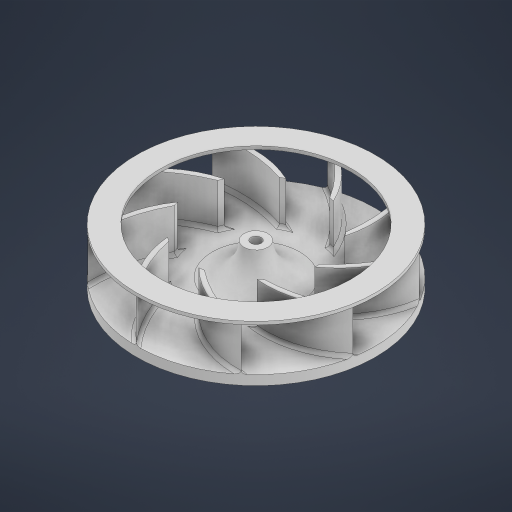
# Autodesk Inventor part: Fan4
Saved by Autodesk Inventor 2023 (Build 270158000, 158)
## iProperties
Created: 2022-10-05
Part Number: Fan4
Material: 一般
Document SubType Name: Modeling
Designer: neko2
Density: 1 g/cm^3
Appearance: 既定
Author: neko2
Autodesk Inventor part; units mm, degrees
ref_plane "YZ Plane" through (0, 0, 0) normal (1, 0, 0) x (0, 1, 0)
ref_plane "XZ Plane" through (0, 0, 0) normal (0, 1, 0) x (-1, 0, 0)
ref_plane "XY Plane" through (0, 0, 0) normal (0, 0, 1) x (1, 0, 0)
sketch "スケッチ1" plane through (0, 0, 0) normal (0, 1, 0) x (-1, 0, 0)
  circle A0 centre (0, 0) radius 7.5
  dimension "d0" = 15
  constraints: 1 centre point, 1 coincident
  measures "d0" diameter of A0
extrude "押し出し1" add sketch "スケッチ1" along normal blind 0.6
sketch "スケッチ2" plane through (0, 0.6, 0) normal (0, 1, 0) x (1, 0, 0)
  circle A0 centre (0, 0) radius 7.5 projected
  circle A1 centre (0, 0) radius 4
  arc A2 (-2, -3.4641) -> (0, -7.5) centre (6.8076, -1.613) ccw
  arc A3 (-2.254, -3.3045) -> (0, -7.5) centre (3.7244, -2.7959) ccw
  dimension "d27" = 8
  dimension "d30" = 9
  dimension "d31" = 6
  dimension "d32" = 0.3
  dimension "d33" = 2
  constraints: 6 point on circle, 3 centre point, 2 vertical alignment, 1 coincident, 1 other
  measures "d27" diameter of A1
  measures "d30" radius of A2
  measures "d31" radius of A3
  measures "d32" distance of A1.start A1.end
  measures "d33" horizontal distance of point (0, 0) A1.start
extrude "押し出し2" add sketch "スケッチ2" along normal blind 2.7 contours A3 A1 A2
fillet "フィレット2" radius 0.2 3 edges at (-1.5611, 0.6, 5.6355) (-1.2566, 0.6, 5.6092) (-2.1285, 0.6, 3.3867)
pattern_circular "円形状パターン3" count 9 over 360 about axis through (0, -10, 0) along (0, 1, 0)
sketch "スケッチ6" plane through (-4.456, 3.3, -1.3534) normal (0, 1, 0) x (0.7460152, 0, 0.665929)
  circle A0 centre (4.2256, 1.9577) radius 6
  circle A1 centre (4.2256, 1.9577) radius 7.5 projected
  circle A2 centre (4.2256, 1.9577) radius 7.5
  dimension "d38" = 1.5
  constraints: 2 centre point, 2 coincident, 1 concentric
  measures "d38" radial gap between concentric circles of A1 A0
extrude "押し出し6" add sketch "スケッチ6" along normal blind 0.2
sketch "スケッチ9" plane through (0, 0.6, 0) normal (0, 1, 0) x (1, 0, 0)
  circle A0 centre (0, 0) radius 0.75
  dimension "d44" = 1.5
  constraints: 1 centre point, 1 coincident
  measures "d44" diameter of A0
extrude "押し出し8" add sketch "スケッチ9" along normal blind 2
fillet "フィレット3" radius 2 1 edges at (-0.75, 0.6, 0)
sketch "スケッチ10" plane through (0, 2.6, 0) normal (0, 1, 0) x (1, 0, 0)
  circle A0 centre (0, 0) radius 0.325
  dimension "d48" = 0.65
  constraints: 1 centre point, 1 coincident
  measures "d48" diameter of A0
extrude "押し出し9" cut sketch "スケッチ10" against normal through all
